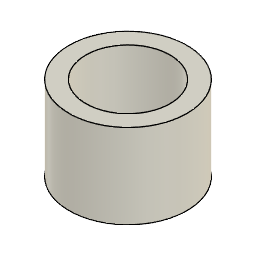
cycloidal_drive (Autodesk Fusion 360 archive; units mm, degrees)
design "entretoise"
Autodesk Fusion 360 part; units mm, degrees
sketch "Esquisse1" plane through (0, 0, 0) normal (0, 0, 1) x (1, 0, 0)
  circle A0 centre (0, 0) radius 2.5
  circle A1 centre (0, 0) radius 3.5
  dimension "d1" = 5
  dimension "d2" = 7
  constraint coincident A0.centre A1.centre
  constraint concentric A0 A1
  measures "d1" diameter of A0
  measures "d2" diameter of A1
extrude "Extrusion1" add sketch "Esquisse1" along normal blind 4
extrude "Extrusion2" add 1 faces at (3.1536, -0.1739, 4) along direction (0, 0, 1) blind 0.5
extrude "Extrusion3" add 1 faces at (3.1536, -0.1739, 0) along direction (0, 0, -1) blind 0.5
